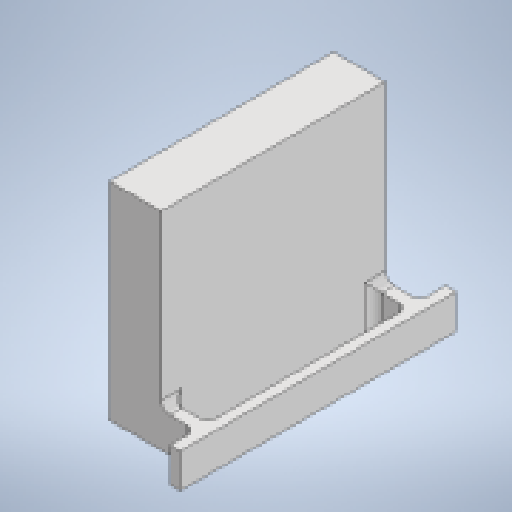
# Autodesk Inventor part: E_box
Saved by Autodesk Inventor 2024 (Build 280153000, 153)
## iProperties
Created: 2023-08-23
Part Number: E_box
Material: Generic
Document SubType Name: Modeling
Designer: l1534
Density: 1 g/cm^3
Appearance: Default
Author: l1534
Autodesk Inventor part; units mm, degrees
ref_plane "YZ Plane" through (0, 0, 0) normal (1, 0, 0) x (0, 1, 0)
ref_plane "XZ Plane" through (0, 0, 0) normal (0, 1, 0) x (-1, 0, 0)
ref_plane "XY Plane" through (0, 0, 0) normal (0, 0, 1) x (1, 0, 0)
sketch "Sketch1" plane through (0, 0, 0) normal (0, 1, 0) x (-1, 0, 0)
  line L0 (3.7362, 151.865) -> (-2.2638, 151.865)
  line L1 (-2.2638, 151.865) -> (-2.2638, -8.135)
  line L2 (-2.2638, -8.135) -> (3.7362, -8.135)
  line L3 (3.7362, -8.135) -> (3.7362, 151.865)
  point P0 (0, 0)
  dimension "d0" = 6
  dimension "d1" = 160
  constraints: 8 end point, 2 parallel, 1 horizontal, 1 perpendicular
  measures "d0" distance of L1.end L2.end
  measures "d1" distance of L2.end L0.start
extrude "Extrusion1" add sketch "Sketch1" along normal blind 20
sketch "Sketch2" plane through (-3.7362, 0, -8.135) normal (-1, 0, 0) x (0, 0, 1)
  line L0 (160, 20) -> (0, 20) projected
  line L1 (15, 20) -> (145, 20)
  line L2 (145, 20) -> (145, 0)
  line L3 (145, 0) -> (15, 0)
  line L4 (15, 0) -> (15, 20)
  line L5 (0, 0) -> (0, 20) projected
  line L6 (160, 0) -> (160, 20) projected
  point P0 (8.135, 0)
  dimension "d4" = 15
  dimension "d5" = 15
  dimension "d6" = 20
  constraints: 8 end point, 2 parallel, 1 horizontal, 1 perpendicular, 1 point on line
  measures "d4" distance between parallel lines of L5 L4
  measures "d5" distance between parallel lines of L6 L2
  measures "d6" distance of L1.end L2.end
extrude "Extrusion2" add sketch "Sketch2" along normal blind 50
sketch "Sketch3" plane through (0, 20, 0) normal (0, 1, 0) x (1, 0, 0)
  line L0 (-3.7362, -136.865) -> (-53.7362, -136.865) projected
  line L1 (-53.7362, -6.865) -> (-23.7362, -6.865)
  line L2 (-23.7362, -6.865) -> (-23.7362, -136.865)
  line L3 (-23.7362, -136.865) -> (-53.7362, -136.865)
  line L4 (-53.7362, -136.865) -> (-53.7362, -6.865)
  point P0 (0, 0)
  dimension "d9" = 30
  constraints: 8 end point, 2 parallel, 1 horizontal, 1 perpendicular, 1 point on line
  measures "d9" distance between parallel lines of L4 L2
extrude "Extrusion3" add sketch "Sketch3" along normal blind 100
sketch "Sketch4" plane through (-3.7362, 0, 6.865) normal (0, 0, -1) x (-1, 0, 0)
  line L0 (50, 0) -> (66, 0)
  line L1 (66, 0) -> (66, 50)
  line L2 (66, 50) -> (50, 50)
  line L3 (50, 50) -> (50, 0)
  point P0 (-3.7362, 0)
  dimension "d12" = 16
  dimension "d13" = 50
  constraints: 8 end point, 2 parallel, 1 horizontal, 1 perpendicular
  measures "d12" distance of L1.end L2.end
  measures "d13" distance of L0.end L1.end
extrude "Extrusion4" add sketch "Sketch4" against normal blind 50
sketch "Sketch6" plane through (0, 20, 0) normal (0, 1, 0) x (1, 0, 0)
  line L0 (-23.7362, -6.865) -> (-23.7362, -136.865) projected
  line L1 (-3.7362, -129.865) -> (-23.7362, -129.865)
  line L2 (-23.7362, -129.865) -> (-23.7362, -13.865)
  line L3 (-23.7362, -13.865) -> (-3.7362, -13.865)
  line L4 (-3.7362, -13.865) -> (-3.7362, -129.865)
  line L5 (-3.7362, -136.865) -> (-23.7362, -136.865) projected
  line L6 (2.2638, -151.865) -> (2.2638, 8.135) projected
  line L7 (-3.7362, -6.865) -> (-23.7362, -6.865) projected
  point P0 (0, 0)
  dimension "d16" = 7
  dimension "d17" = 6
  dimension "d18" = 7
  constraints: 8 end point, 2 parallel, 1 horizontal, 1 perpendicular, 1 point on line
  measures "d16" distance between parallel lines of L5 L1
  measures "d17" distance between parallel lines of L6 L4
  measures "d18" distance between parallel lines of L7 L3
extrude "Extrusion5" cut sketch "Sketch6" against normal blind 50
fillet "Fillet1" radius 5 4 edges at (-23.7362, 20, 133.365) (-23.7362, 20, 10.365) (-23.7362, 10, 129.865) (-23.7362, 10, 13.865)
fillet "Fillet2" radius 5 4 edges at (-3.7362, 10, 129.865) (-3.7362, 10, 13.865) (-3.7362, 10, 6.865) (-3.7362, 10, 136.865)
body "Solid1"
